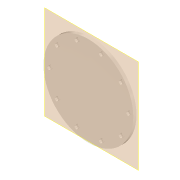
# Autodesk Inventor part: Anglerfish_Frontwindow_v0
Saved by Autodesk Inventor 2022 (Build 260153000, 153)
## iProperties
Created: 2022-04-02
Part Number: Anglerfish_Frontwindow_v0
Material: Generic
Document SubType Name: Modeling
Designer: Prakash Lab
Density: 1 g/cm^3
Appearance: Polycarbonate - Clear
Author: Prakash Lab
Autodesk Inventor part; units mm, degrees
ref_plane "YZ Plane" through (0, 0, 0) normal (1, 0, 0) x (0, 1, 0)
ref_plane "XZ Plane" through (0, 0, 0) normal (0, 1, 0) x (-1, 0, 0)
ref_plane "XY Plane" through (0, 0, 0) normal (0, 0, 1) x (1, 0, 0)
ref_plane "Work Plane1" through (0, 0, 0) normal (0, 0, 1) x (1, 0, 0)
sketch "Sketch1" plane through (0, 0, 0) normal (0, 0, 1) x (1, 0, 0)
  circle A0 centre (0, 0) radius 40 projected
  circle A1 centre (0, 0) radius 40 projected
  circle A2 centre (37, 0) radius 1.4 projected
  circle A3 centre (29.9336, 21.7481) radius 1.4 projected
  circle A4 centre (11.4336, 35.1891) radius 1.4 projected
  circle A5 centre (-11.4336, 35.1891) radius 1.4 projected
  circle A6 centre (-29.9336, 21.7481) radius 1.4 projected
  circle A7 centre (-37, 0) radius 1.4 projected
  circle A8 centre (-29.9336, -21.7481) radius 1.4 projected
  circle A9 centre (-11.4336, -35.1891) radius 1.4 projected
  circle A10 centre (11.4336, -35.1891) radius 1.4 projected
  circle A11 centre (29.9336, -21.7481) radius 1.4 projected
  circle A12 centre (0, 0) radius 34 projected
  circle A13 centre (0, 0) radius 42
  point P0 (0, 0)
  dimension "d9" = 2
  constraints: 1 centre point
  measures "d9" radial gap between concentric circles of A0 A13
extrude "Extrusion1" add sketch "Sketch1" along normal blind 3 contours A0 | A12
sketch "Sketch2" plane through (0, 0, 3) normal (0, 0, 1) x (1, 0, 0)
  circle A0 centre (0, 0) radius 40 projected
  circle A1 centre (29.9336, -21.7481) radius 1.4 projected
  circle A2 centre (11.4336, -35.1891) radius 1.4 projected
  circle A3 centre (-11.4336, -35.1891) radius 1.4 projected
  circle A4 centre (-29.9336, -21.7481) radius 1.4 projected
  circle A5 centre (-37, 0) radius 1.4 projected
  circle A6 centre (-29.9336, 21.7481) radius 1.4 projected
  circle A7 centre (-11.4336, 35.1891) radius 1.4 projected
  circle A8 centre (11.4336, 35.1891) radius 1.4 projected
  circle A9 centre (29.9336, 21.7481) radius 1.4 projected
  circle A10 centre (37, 0) radius 1.4 projected
  point P0 (0, 0)
hole "Hole1" at (29.9336, 21.7481, 3) at (37, 0, 3) at (29.9336, -21.7481, 3) at (11.4336, -35.1891, 3) at (-11.4336, -35.1891, 3) at (-29.9336, -21.7481, 3) at (-37, 0, 3) at (-29.9336, 21.7481, 3) at (-11.4336, 35.1891, 3) at (11.4336, 35.1891, 3) direction (0, 0, -1) diameter 3.1 end through all
sketch "Sketch3" plane through (0, 0, 3) normal (0, 0, 1) x (1, 0, 0)
  circle A0 centre (0, 0) radius 40 projected
  circle A1 centre (0, 0) radius 42
  point P0 (0, 0)
  dimension "d10" = 2
  constraints: 1 centre point
  measures "d10" radial gap between concentric circles of A0 A1
ref_plane "Work Plane2" through (-40, -40, 0) normal (0, 0, 1) x (1, 0, 0)
extrude "Extrusion2" add sketch "Sketch3" against normal up to surface (3 mm away)
body "Solid1"
